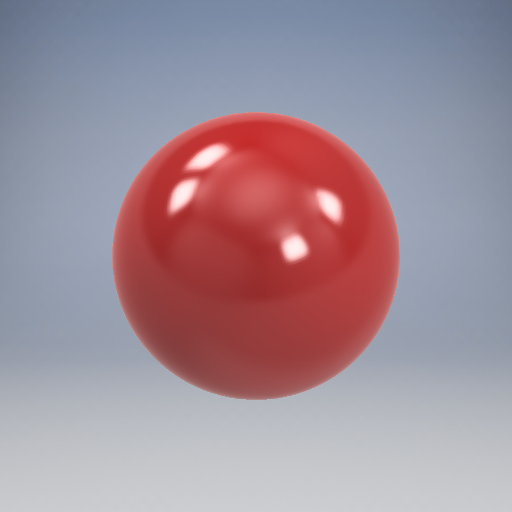
# Autodesk Inventor part: ball
Saved by Autodesk Inventor 2025.3 (Build 293356000, 356)
## iProperties
Created: 2026-02-27
Part Number: ball
Material: PPS Plastic
Document SubType Name: Modeling
Designer: user
Density: 1.637 g/cm^3
Appearance: Red
Mass: 23.1425 g
Surface Area: 28.2743 cm^2
Volume: 14.1372 cm^3
Author: user
Autodesk Inventor part; units mm, degrees
ref_plane "YZ Plane" through (0, 0, 0) normal (1, 0, 0) x (0, 1, 0)
ref_plane "XZ Plane" through (0, 0, 0) normal (0, 1, 0) x (-1, 0, 0)
ref_plane "XY Plane" through (0, 0, 0) normal (0, 0, 1) x (1, 0, 0)
sketch "Sketch1" plane through (0, 0, 0) normal (0, 1, 0) x (-1, 0, 0)
  arc A0 (-15, 0) -> (15, 0) centre (0, 0) ccw
  line L0 (15, 0) -> (-15, 0)
  dimension "d0" = 30
  dimension "d1" = 30
  constraints: 2 end point, 2 point on circle, 1 centre point, 1 coincident, 1 horizontal
  measures "d0" diameter of A0
  measures "d1" distance of L0.start L0.end
revolve "Revolution1" add sketch "Sketch1" angle 360 about axis through (-15, 0, 0) along (1, 0, 0)
body "Solid1"
